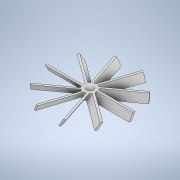
# Autodesk Inventor part: AERO - Propeller
Saved by Autodesk Inventor 2021 (Build 250183000, 183)
## iProperties
Created: 2021-01-21
Part Number: AERO - Propeller
Material: Generic
Document SubType Name: Modeling
Designer: garciar1
Density: 1 g/cm^3
Appearance: Default
Author: garciar1
Autodesk Inventor part; units mm, degrees
ref_plane "YZ Plane" through (0, 0, 0) normal (1, 0, 0) x (0, 1, 0)
ref_plane "XZ Plane" through (0, 0, 0) normal (0, 1, 0) x (-1, 0, 0)
ref_plane "XY Plane" through (0, 0, 0) normal (0, 0, 1) x (1, 0, 0)
sketch "Sketch1" plane through (0, 0, 0) normal (0, 1, 0) x (-1, 0, 0)
  circle A0 centre (0, 0) radius 10
  dimension "d0" = 20
  constraints: 1 centre point, 1 coincident
  measures "d0" diameter of A0
extrude "Extrusion1" add sketch "Sketch1" along normal blind 10
sketch "Sketch3" plane through (0, 0, 0) normal (1, 0, 0) x (0, 1, 0)
  line L0 (0, 5) -> (10, -0.7735)
  line L1 (10, -0.7735) -> (10, -3.7735)
  line L2 (10, -3.7735) -> (0, 2)
  line L3 (0, 2) -> (0, 5)
  point P0 (0, 0)
  dimension "d3" = 3
  dimension "d4" = 10
  dimension "d5" = 10
  dimension "d6" = 60
  dimension "d7" = 5
  constraints: 8 end point, 2 parallel, 1 vertical
  measures "d3" distance of L0.end L1.end
  measures "d4" horizontal distance of point (0, 0) L1.end
  measures "d5" horizontal distance of L0.start L0.end
  measures "d6" angle of L3 L0
  measures "d7" distance of point (0, 0) L0.start
extrude "Extrusion2" add sketch "Sketch3" along normal blind 63.5
pattern_circular "Circular Pattern1" count 10 over 360 about axis through (0, 0, 0) along (0, 1, 0) of "Extrusion2"
sketch "Sketch4" plane through (0, 10, 0) normal (0, 1, 0) x (1, 0, 0)
  circle A0 centre (0, 0) radius 5
  dimension "d13" = 10
  constraints: 1 centre point, 1 coincident
  measures "d13" diameter of A0
extrude "Extrusion3" add sketch "Sketch4" along normal blind 5
fillet "Fillet1" radius 5 1 edges at (-5, 15, 0)
sketch "Sketch5" plane through (0, 0, 0) normal (0, -1, 0) x (1, 0, 0)
  circle A0 centre (0, 0) radius 2.5
  dimension "d17" = 5
  constraints: 1 centre point, 1 coincident
  measures "d17" diameter of A0
extrude "Extrusion4" cut sketch "Sketch5" against normal blind 2
body "Solid1"
